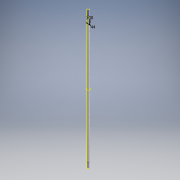
# Autodesk Inventor part: PipeB
Saved by Autodesk Inventor 2017 (Build 210142000, 142)
## iProperties
Created: 2017-10-25
Part Number: PipeB
Material: Generic
Document SubType Name: Modeling
Designer: Hor
Density: 1 g/cm^3
Appearance: Default
Author: Hor
Autodesk Inventor part; units mm, degrees
sketch "Sketch1" plane through (0, 0, 0) normal (0, 0, 1) x (1, 0, 0)
  circle A0 centre (0, 0) radius 38
  circle A1 centre (0, 0) radius 36
  dimension "d0" = 76
  dimension "d1" = 72
  constraints: 2 centre point, 2 coincident
  measures "d0" diameter of A0
  measures "d1" diameter of A1
extrude "Extrusion1" add sketch "Sketch1" along normal blind 2000 and the other way blind 2000
sketch "Sketch2" plane through (0, 0, 0) normal (0, 1, 0) x (-1, 0, 0)
  line L0 (-38, -2000) -> (38, -2000) projected
  line L1 (38, 2000) -> (-38, 2000) projected
  line L2 (38, 2000) -> (-38, 2000) projected
  circle A0 centre (0, 1800) radius 22
  point P0 (0, 0)
  point P1 (0, -2000)
  dimension "d4" = 44
  dimension "d18" = 200
  constraints: 1 centre point, 1 midpoint, 1 vertical alignment
  measures "d4" diameter of A0
  measures "d18" distance from line of L1 A0.centre
extrude "Extrusion2" cut sketch "Sketch2" along normal through all
pattern_linear "Rectangular Pattern1" count 19 spacing 200 along (0, 0, -1) of "Extrusion2"
body "Solid1"
